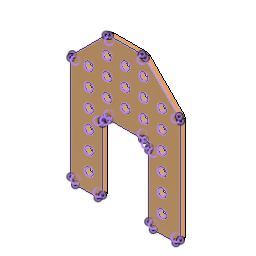
Custom U-Bracket (Autodesk Fusion 360 design; units mm, degrees)
Autodesk Fusion 360 part; units mm, degrees
sketch "Sketch1" plane through (0, 0, 0) normal (0, 1, 0) x (1, 0, 0)
  line L0 (0, 0) -> (0, -76.2)
  line L1 (0, -76.2) -> (76.2, -76.2)
  line L2 (76.2, -76.2) -> (76.2, 0)
  line L3 (76.2, 0) -> (54.102, 0)
  line L4 (54.102, 0) -> (54.102, -50.8)
  line L5 (54.102, -50.8) -> (22.098, -50.8)
  line L6 (22.098, -50.8) -> (22.098, 0)
  line L7 (22.098, 0) -> (0, 0)
  line L8 (12.7, 0) -> (12.7, -76.2) construction
  line L9 (38.1, -50.8) -> (38.1, -76.2) construction
  circle A0 centre (23.7818, -49.1162) radius 2.3813
  line L10 (23.7818, -49.1162) -> (23.7818, -50.8) construction
  line L11 (23.7818, -49.1162) -> (22.098, -49.1162) construction
  circle A1 centre (12.7, -12.7) radius 2.7781
  circle A2 centre (12.7, -25.4) radius 2.7781
  line L12 (12.7, -12.7) -> (12.7, -88.9) construction
  circle A3 centre (12.7, -38.1) radius 2.7781
  line L13 (12.7, -25.4) -> (12.7, -101.6) construction
  circle A4 centre (12.7, -50.8) radius 2.7781
  line L14 (12.7, -38.1) -> (12.7, -114.3) construction
  circle A5 centre (12.7, -63.5) radius 2.7781
  line L15 (12.7, -50.8) -> (12.7, -127) construction
  circle A6 centre (63.5, -38.1) radius 2.7781
  circle A7 centre (63.5, -50.8) radius 2.7781
  circle A8 centre (63.5, -63.5) radius 2.7781
  circle A9 centre (63.5, -25.4) radius 2.7781
  circle A10 centre (63.5, -12.7) radius 2.7781
  circle A11 centre (52.4182, -49.1162) radius 2.3813
  circle A12 centre (38.1, -63.5) radius 2.7781
  line L16 (0, -76.2) -> (25.4, -101.6)
  line L17 (25.4, -101.6) -> (50.8, -101.6)
  line L18 (50.8, -101.6) -> (76.2, -76.2)
  circle A13 centre (38.1, -76.2) radius 2.7781
  circle A14 centre (38.1, -88.9) radius 2.7781
  circle A15 centre (25.4, -63.5) radius 2.7781
  circle A16 centre (25.4, -76.2) radius 2.7781
  circle A17 centre (25.4, -88.9) radius 2.7781
  circle A18 centre (12.7, -76.2) radius 2.7781
  circle A19 centre (50.8, -63.5) radius 2.7781
  circle A20 centre (50.8, -76.2) radius 2.7781
  circle A21 centre (50.8, -88.9) radius 2.7781
  circle A22 centre (63.5, -76.2) radius 2.7781
  dimension "d1" = 76.2
  dimension "d3" = 32.004
  dimension "d4" = 50.8
  dimension "d6" = 76.2
  dimension "d7" = 12.7
  dimension "d8" = 4.7625
  dimension "d9" = 5.5563
  dimension "d10" = 12.7
  dimension "d13" = 0
  dimension "d14" = -50.8
  dimension "d17" = 25.4
  dimension "d18" = 0
  dimension "d25" = 25.4
  dimension "d26" = 25.4
  dimension "d29" = 25.4
  dimension "d30" = 0
  dimension "d33" = 12.7
  dimension "d34" = 0
  dimension "d37" = 0
  dimension "d38" = -25.4
  dimension "d41" = 0
  dimension "d42" = -12.7
  constraint coincident L0.start L7.end
  constraint vertical L0
  constraint perpendicular L0 L1
  constraint perpendicular L1 L2
  constraint perpendicular L2 L3
  constraint perpendicular L3 L4
  constraint perpendicular L4 L5
  constraint perpendicular L5 L6
  constraint perpendicular L0 L7
  constraint equal L3 L7
  constraint coincident L1 L8.end
  constraint perpendicular L1 L8
  constraint midpoint L5 L9.start
  constraint midpoint L1 L9.end
  constraint coincident L7 L8.start
  constraint equal L0 L2
  constraint coincident L5.end A0
  constraint coincident A0.centre L10.start
  constraint coincident L5 L10.end
  constraint perpendicular L5 L10
  constraint coincident L6 L11.end
  constraint perpendicular L6 L11
  constraint equal L10 L11
  constraint coincident L8 A1.centre
  constraint symmetric L9 A0 A11
  constraint symmetric L9 A1 A10
  constraint symmetric L9 A2 A9
  constraint symmetric L9 A3 A6
  constraint symmetric L9 A4 A7
  constraint symmetric L9 A5 A8
  constraint perpendicular L0 L17
  constraint equal L16 L18
  constraint symmetric L9 A15 A19
  constraint symmetric L9 A16 A20
  constraint symmetric L9 A17 A21
  constraint symmetric L9 A18 A22
  measures "d1" distance of L0 L2
  measures "d3" distance of L4.end L5.end
  measures "d4" distance of L5.end L6.end
  measures "d6" distance of L0.start L0.end
  measures "d7" distance of L0 L8
  measures "d8" diameter of A0
  measures "d9" diameter of A1
  measures "d10" distance of L7 A1.centre
  measures "d25" distance of L1 L17
  measures "d26" distance of L16.end L17.end
extrude "Extrude1" add sketch "Sketch1" along normal blind 3.175 contours L0 L1 L2 L3 L4 L5 L6 L7 A0 A11 A13 A16 A18 A20 A22 | L1 L16 L17 L18 A13 A16 A18 A20 A22
fillet "Fillet1" radius 3.175 8 edges at (0, 1.5875, 0) (22.098, 1.5875, 0) (54.102, 1.5875, 0) (76.2, 1.5875, 0) (0, 1.5875, 76.2) (25.4, 1.5875, 101.6) (50.8, 1.5875, 101.6) (76.2, 1.5875, 76.2)
fillet "Fillet1" radius 3.175 4 edges at (25.4656, 1.5875, 50.8) (22.098, 1.5875, 47.4324) (50.7344, 1.5875, 50.8) (54.102, 1.5875, 47.4324)
sketch "DXF" plane through (0, 0, 0) normal (0, -1, 0) x (1, 0, 0)
  circle A0 centre (38.1, 76.2) radius 2.7781
  circle A1 centre (25.4, 76.2) radius 2.7781
  circle A2 centre (63.5, 12.7) radius 2.7781
  circle A3 centre (63.5, 25.4) radius 2.7781
  circle A4 centre (63.5, 63.5) radius 2.7781
  circle A5 centre (63.5, 50.8) radius 2.7781
  circle A6 centre (63.5, 38.1) radius 2.7781
  circle A7 centre (12.7, 63.5) radius 2.7781
  circle A8 centre (12.7, 12.7) radius 2.7781
  circle A9 centre (12.7, 25.4) radius 2.7781
  circle A10 centre (12.7, 38.1) radius 2.7781
  circle A11 centre (12.7, 50.8) radius 2.7781
  circle A12 centre (63.5, 76.2) radius 2.7781
  circle A13 centre (25.4, 63.5) radius 2.7781
  circle A14 centre (25.4, 88.9) radius 2.7781
  circle A15 centre (38.1, 88.9) radius 2.7781
  circle A16 centre (50.8, 76.2) radius 2.7781
  circle A17 centre (38.1, 63.5) radius 2.7781
  circle A18 centre (12.7, 76.2) radius 2.7781
  circle A19 centre (50.8, 88.9) radius 2.7781
  circle A20 centre (50.8, 63.5) radius 2.7781
  arc A21 (54.5005, 47.9611) -> (54.102, 46.421) centre (57.277, 46.421) ccw
  line L0 (54.102, 46.421) -> (54.102, 3.175)
  arc A22 (54.102, 3.175) -> (57.277, 0) centre (57.277, 3.175) ccw
  line L1 (57.277, 0) -> (73.025, 0)
  arc A23 (73.025, 0) -> (76.2, 3.175) centre (73.025, 3.175) ccw
  line L2 (76.2, 3.175) -> (76.2, 74.8849)
  arc A24 (76.2, 74.8849) -> (75.2701, 77.1299) centre (73.025, 74.8849) ccw
  line L3 (75.2701, 77.1299) -> (51.7299, 100.6701)
  arc A25 (51.7299, 100.6701) -> (49.4849, 101.6) centre (49.4849, 98.425) ccw
  line L4 (49.4849, 101.6) -> (26.7151, 101.6)
  arc A26 (26.7151, 101.6) -> (24.4701, 100.6701) centre (26.7151, 98.425) ccw
  line L5 (24.4701, 100.6701) -> (0.9299, 77.1299)
  arc A27 (0.9299, 77.1299) -> (0, 74.8849) centre (3.175, 74.8849) ccw
  line L6 (0, 74.8849) -> (0, 3.175)
  arc A28 (0, 3.175) -> (3.175, 0) centre (3.175, 3.175) ccw
  line L7 (3.175, 0) -> (18.923, 0)
  arc A29 (18.923, 0) -> (22.098, 3.175) centre (18.923, 3.175) ccw
  line L8 (22.098, 3.175) -> (22.098, 46.421)
  arc A30 (22.098, 46.421) -> (21.6995, 47.9611) centre (18.923, 46.421) ccw
  arc A31 (24.9369, 51.1985) -> (21.6995, 47.9611) centre (23.7818, 49.1162) ccw
  arc A32 (24.9369, 51.1985) -> (26.477, 50.8) centre (26.477, 53.975) ccw
  line L9 (26.477, 50.8) -> (49.723, 50.8)
  arc A33 (49.723, 50.8) -> (51.2631, 51.1985) centre (49.723, 53.975) ccw
  arc A34 (54.5005, 47.9611) -> (51.2631, 51.1985) centre (52.4182, 49.1162) ccw
equation "TOLERANCE = 0.01 in" comment "Tube size tolerance"
equation "d3 = 1 in + 2 * BRACKET_THICKNESS + TOLERANCE"
equation "d9 = HOLE_DIAMETER"
equation "HOLE_DIAMETER = ( 7 / 32 ) * 1 in"
equation "BRACKET_THICKNESS = ( 1 / 8 ) * 1 in" comment "Thickness of the bracket"
